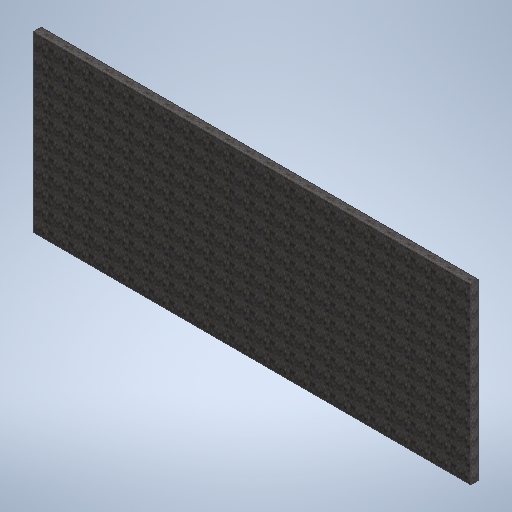
# Autodesk Inventor part: Wand
Saved by Autodesk Inventor 2025.1 (Build 291241000, 241)
## iProperties
Created: 2024-08-07
Part Number: Wand
Material: Concrete
Document SubType Name: Modeling
Designer: ffogue
Density: 2.40731 g/cm^3
Appearance: Exposed Aggregate - Coarse
Author: ffogue
Autodesk Inventor part; units mm, degrees
ref_plane "YZ Plane" through (0, 0, 0) normal (1, 0, 0) x (0, 1, 0)
ref_plane "XZ Plane" through (0, 0, 0) normal (0, 1, 0) x (-1, 0, 0)
ref_plane "XY Plane" through (0, 0, 0) normal (0, 0, 1) x (1, 0, 0)
sketch "Sketch1" plane through (0, 0, 0) normal (0, 0, 1) x (1, 0, 0)
  line L0 (0, 0) -> (5000, 0)
  line L1 (5000, 0) -> (5000, 90)
  line L2 (5000, 90) -> (0, 90)
  line L3 (0, 90) -> (0, 0)
  dimension "d0" = 90
  dimension "d1" = 5000
  constraints: 8 end point, 2 parallel, 1 horizontal, 1 perpendicular
  measures "d0" distance between parallel lines of L0 L2
  measures "d1" distance of L1.end L2.end
extrude "Extrusion1" add sketch "Sketch1" along normal blind 1985
body "Solid1"
